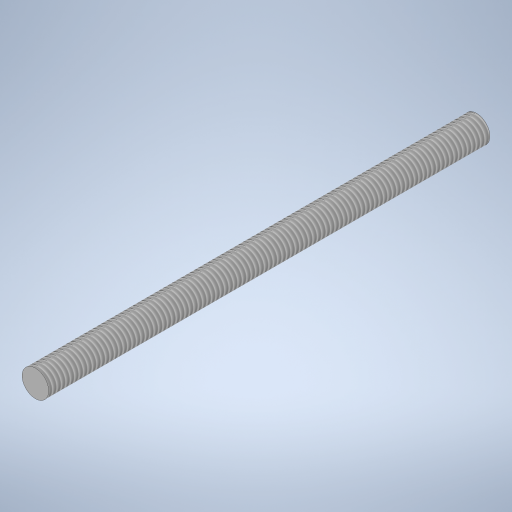
# Autodesk Inventor part: Axle
Saved by Autodesk Inventor 2024.3 (Build 283343000, 343)
## iProperties
Created: 2024-11-27
Part Number: Axle
Material: Generisch
Document SubType Name: Modeling
Designer: Maximilian Hock
Density: 1 g/cm^3
Appearance: Vorgabe
Author: Maximilian Hock
Autodesk Inventor part; units mm, degrees
ref_plane "YZ Plane" through (0, 0, 0) normal (1, 0, 0) x (0, 1, 0)
ref_plane "XZ Plane" through (0, 0, 0) normal (0, 1, 0) x (-1, 0, 0)
ref_plane "XY Plane" through (0, 0, 0) normal (0, 0, 1) x (1, 0, 0)
sketch "Skizze1" plane through (0, 0, 0) normal (0, 1, 0) x (-1, 0, 0)
  circle A0 centre (0, 0) radius 3
  dimension "d0" = 6
  constraints: 1 centre point, 1 coincident
  measures "d0" diameter of A0
extrude "Extrusion1" add sketch "Skizze1" along normal blind 100
thread "Gewinde1" size "M6x1" class "6g" standard "ANSI Metric M Profile" full length
equation "\"d0\" = AxleDiameter"
equation "\"d1\" = AxleLength"
equation "\"AxleDiameter\" = 6"
equation "\"AxleLength\" = 100"
